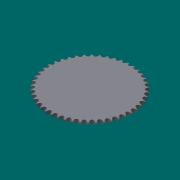
# Autodesk Inventor part: Roller Chain Sprocket1
Saved by Autodesk Inventor 2016 (Build 200138000, 138)
## iProperties
Created: 2017-01-14
Part Number: Roller Chain Sprocket1
Material: Steel
Document SubType Name: Modeling
Designer: katzchristy
Density: 1 g/cm^3
Appearance: Steel
CustomPartVersion: 1
Author: katzchristy
Autodesk Inventor part; units mm, degrees
ref_plane "YZ Plane" through (0, 0, 0) normal (1, 0, 0) x (0, 1, 0)
ref_plane "XZ Plane" through (0, 0, 0) normal (0, 1, 0) x (-1, 0, 0)
sketch "Theoretical Tooth Profile" plane through (0, 0, 0) normal (0, 0, 1) x (1, 0, 0)
  circle A0 centre (0, 0) radius 93.0506 construction
  line L0 (0, 0) -> (0, 93.0506) construction
  line L1 (0, 0) -> (12.6704, 92.184) construction
  circle A1 centre (0, 0) radius 96.6437
  arc A2 (-3.154, 90.7334) -> (3.154, 90.7334) centre (0, 93.0506) ccw
  line L2 (0, 93.0506) -> (12.6704, 92.184) construction
  line L3 (0, 93.0506) -> (4.9965, 96.7215) construction
  line L4 (4.9965, 96.7215) -> (-4.5359, 93.3418) construction
  arc A3 (6.1131, 96.4502) -> (4.9132, 94.4061) centre (10.8247, 92.3102) ccw
  arc A4 (-4.9132, 94.4061) -> (-6.1131, 96.4502) centre (-10.8247, 92.3102) ccw
  line L5 (-10.8247, 92.3102) -> (-4.9132, 94.4061) construction
  arc A5 (-4.5359, 93.3418) -> (-3.154, 90.7334) centre (4.9965, 96.7215) ccw
  line L6 (-4.5359, 93.3418) -> (-4.9132, 94.4061)
  arc A6 (3.154, 90.7334) -> (4.5359, 93.3418) centre (-4.9965, 96.7215) ccw
  line L7 (4.9132, 94.4061) -> (4.5359, 93.3418)
  line L8 (0, 0) -> (6.5952, 96.4184) construction
  point P0 (6.3352, 92.6173)
  dimension "d0" = 186.1013
  dimension "d2" = 7.826
  dimension "d3" = 3.9137
  dimension "d10" = 126.304
  dimension "d11" = 16.783
  dimension "d12" = 6.2
  dimension "d13" = 10.1137
  dimension "d14" = 10.85
  dimension "d23" = 3.81
  constraints: 18 end point, 15 point on circle, 7 centre point, 3 coincident, 3 point on line, 3 symmetric about line, 3 tangent, 1 equal radius, 1 midpoint, 1 parallel, 1 vertical, 1 other
  measures "d0" diameter of A0
  measures "d2" angle of L1 L0
  measures "d3" radius of A2
  measures "d10" angle of L3 L0
  measures "d11" angle of L4 L3
  measures "d12" distance of L2.start L3.end
  measures "d13" distance of L3.end L4.end
  measures "d14" distance of A3.centre L0.end
  measures "d23" distance from line of L8.end L2
sketch "Tooth Profile" plane through (0, 0, 0) normal (0, 0, 1) x (1, 0, 0)
  circle A0 centre (0, 0) radius 96.6437 projected
  line L0 (0, 0) -> (0, 93.0506) construction
  line L1 (0, 93.0506) -> (3.6543, 91.6495) construction
  arc A1 (-3.6543, 91.6495) -> (3.6543, 91.6495) centre (0, 93.0506) ccw
  line L2 (-3.6543, 91.6495) -> (0, 93.0506) construction
  arc A2 (-3.6543, 91.6495) -> (-5.8372, 96.4673) centre (-45.3354, 75.6677) ccw
  arc A3 (5.8372, 96.4673) -> (3.6543, 91.6495) centre (45.3354, 75.6677) ccw
  dimension "d44" = 138.043
  dimension "d45" = 3.9137
  dimension "d46" = 44.64
  constraints: 8 point on circle, 7 end point, 3 centre point, 2 tangent, 1 coincident, 1 equal radius, 1 symmetric about line, 1 vertical
  measures "d44" angle of L1 L2
  measures "d45" radius of A1
  measures "d46" radius of A3
sketch "Section Profile" plane through (0, 0, 0) normal (1, 0, 0) x (0, 1, 0)
  line L0 (96.6437, 0) -> (-96.6437, 0) projected
  line L1 (83.3725, 1.5345) -> (-83.3725, 1.5345)
  line L2 (-83.3725, 1.5345) -> (-83.3725, -1.5345)
  line L3 (-83.3725, -1.5345) -> (83.3725, -1.5345)
  line L4 (83.3725, -1.5345) -> (83.3725, 1.5345)
  line L5 (83.3725, 1.5345) -> (96.6437, 1.5345) construction
  line L6 (96.6437, 1.5345) -> (96.6437, -1.5345) construction
  line L7 (96.6437, -1.5345) -> (83.3725, -1.5345) construction
  line L8 (83.3725, -1.5345) -> (83.3725, 1.5345)
  arc A0 (96.6437, 0.7725) -> (92.3108, 1.5345) centre (92.3108, -11.1655) ccw
  arc A1 (92.3108, -1.5345) -> (96.6437, -0.7725) centre (92.3108, 11.1655) ccw
  line L9 (92.3108, 1.5345) -> (0, 1.5345)
  line L10 (0, 1.5345) -> (0, -1.5345)
  line L11 (0, -1.5345) -> (92.3108, -1.5345)
  line L12 (0, 1.5345) -> (0, -1.5345)
  line L13 (96.6437, 0.7725) -> (96.6437, -0.7725)
  point P0 (0, 0)
  point P1 (0, 0)
  dimension "d30" = 3.069
  dimension "d31" = 166.745
  dimension "d32" = 3.069
  dimension "d33" = 0.762
  dimension "d34" = 12.7
  dimension "d43" = 1.5345
  constraints: 26 end point, 7 midpoint, 5 perpendicular, 4 parallel, 4 point on circle, 3 point on line, 3 symmetric about line, 2 centre point, 2 horizontal, 2 tangent, 1 collinear, 1 other
  measures "d30" distance between parallel lines of L7 L5
  measures "d31" distance between parallel lines of L2 L4
  measures "d32" distance between parallel lines of L3 L1
  measures "d33" distance from line of L13.start L5
  measures "d34" radius of A0
  measures "d43" distance between parallel lines of L3 L0
revolve "Shroud" add sketch "Section Profile" angle 360 about axis through (0, 0, 1.5345) along (0, 0, -1) contours L10 L3 L2 L0 | L0 L2 L1 L10
revolve "Strand" add sketch "Section Profile" angle 360 about axis through (0, 0, 1.5345) along (0, 0, -1) contours L13 A1 L11 L4 L0 | L0 L4 L9 A0 L13 | L4 L3 L10 L0 | L0 L10 L1 L4
pattern_of_one "Strand Pattern"
extrude "Theoretical Tooth" cut sketch "Theoretical Tooth Profile" along normal through all both and the other way through all contours A3 L7 A6 A2 A5 L6 A4 A1 picked at (0.6796, 92.6963)
extrude "Tooth" [suppressed]
pattern_circular "Tooth Pattern" count 46 over 360 about axis through (0, 0, -10) along (0, 0, 1) of "Theoretical Tooth"
ref_plane "Timing Plane" through (0, 93.0506, 0) normal (1, 0, 0) x (0, 1, 0)
equation "\"d3\" = 0.5 * da_Dr + da_SC"
equation "\"d12\" = 0.8 * da_Dr"
equation "\"d13\" = 1.3 * da_Dr + da_SC"
equation "\"d14\" = 1.4 * da_Dr"
equation "\"d23\" = da_Ha"
equation "\"d44\" = da_Alfa"
equation "\"d45\" = da_Ri"
equation "\"d46\" = da_Re"
equation "\"d30\" = da_Bf"
equation "\"d31\" = da_Ds"
equation "\"d32\" = da_Bs"
equation "\"d33\" = da_Ba"
equation "\"d34\" = da_Rx"
equation "\"d40\" = da_pt"
equation "\"form_type\" = 0"
equation "\"da_p\" = 12.7"
equation "\"da_Dr\" = 7.75"
equation "\"da_SC\" = 0.03875"
equation "\"da_Ha\" = 3.81"
equation "\"da_pt\" = 13.92"
equation "\"da_Bf\" = 3.069"
equation "\"da_Ba\" = 0.762"
equation "\"da_Rx\" = 12.7"
equation "\"da_Ra\" = 0.508"
equation "\"da_Bs\" = 3.069"
equation "\"da_Ds\" = 166.74503"
equation "\"da_Re\" = 44.64"
equation "\"da_Ri\" = 3.91375"
equation "\"da_Alfa\" = 138.043deg"
body "Solid1"
